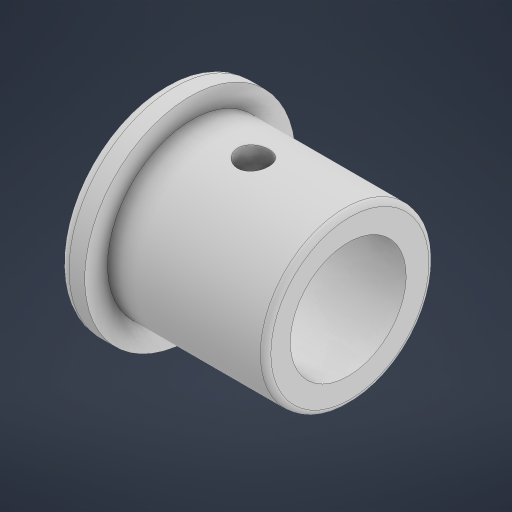
# Autodesk Inventor part: sf_Crankshaft_Bearing_Bush_1
Saved by Autodesk Inventor 2024 (Build 280153000, 153)
## iProperties
Created: 2024-03-20
Part Number: sf_Crankshaft_Bearing_Bush_1
Material: Generisch
Document SubType Name: Modeling
Designer: Simon
Density: 1 g/cm^3
Appearance: Vorgabe
Author: Simon
Autodesk Inventor part; units mm, degrees
ref_plane "YZ Plane" through (0, 0, 0) normal (1, 0, 0) x (0, 1, 0)
ref_plane "XZ Plane" through (0, 0, 0) normal (0, 1, 0) x (-1, 0, 0)
ref_plane "XY Plane" through (0, 0, 0) normal (0, 0, 1) x (1, 0, 0)
sketch "Skizze1" plane through (0, 0, 0) normal (1, 0, 0) x (0, 1, 0)
  circle A0 centre (0, 0) radius 10
  dimension "d0" = 20
  constraints: 1 centre point, 1 coincident
  measures "d0" diameter of A0
extrude "Extrusion1" add sketch "Skizze1" along normal blind 2.5
sketch "Skizze2" plane through (2.5, 0, 0) normal (1, 0, 0) x (0, 0, -1)
  circle A0 centre (0, 0.1551) radius 7.9987
  circle A1 centre (0, 0) radius 5.5
  dimension "d3" = 15.9975
  dimension "d4" = 11
  constraints: 2 centre point, 1 coincident
  measures "d3" diameter of A0
  measures "d4" diameter of A1
extrude "Extrusion2" add sketch "Skizze2" along normal blind 15
sketch "Skizze3" plane through (0, 0, 0) normal (0, 0, 1) x (1, 0, 0)
  circle A0 centre (8.5, 0) radius 1.5
  point P0 (0, 0)
  dimension "d7" = 3
  constraints: 1 centre point
  measures "d7" diameter of A0
extrude "Extrusion3" cut sketch "Skizze3" along normal up to surface round surface about axis through (2.5, 0.1551, 0) along (1, 0, 0) radius 7.9987 far side no
fillet "Rundung1" radius 0.5 1 edges at (17.5, 0.1551, 7.9987)
fillet "Rundung2" radius 1 1 edges at (0, -10, 0)
delete faces "Fläche löschen1" heal yes whole lump no faces at (2.5, 0.4132, -1.5701)
